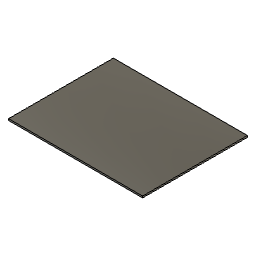
2nd Plate M v6 (Autodesk Fusion 360 design; units mm, degrees)
Autodesk Fusion 360 part; units mm, degrees
sketch "Sketch1" plane through (0, 0, 0) normal (0, 0, 1) x (1, 0, 0)
  line L0 (-250, 225) -> (180, 225)
  line L1 (180, 225) -> (180, -111.4)
  line L2 (180, -111.4) -> (-250, -111.4)
  line L3 (-250, -111.4) -> (-250, 225)
  dimension "d1" = 336.4
  dimension "d2" = 430
  constraint horizontal L0
  constraint vertical L1
  constraint horizontal L2
  constraint vertical L3
  measures "d1" distance of L0.start L2.end
  measures "d2" distance of L0.start L0.end
extrude "Extrude1" add sketch "Sketch1" along normal blind 5
